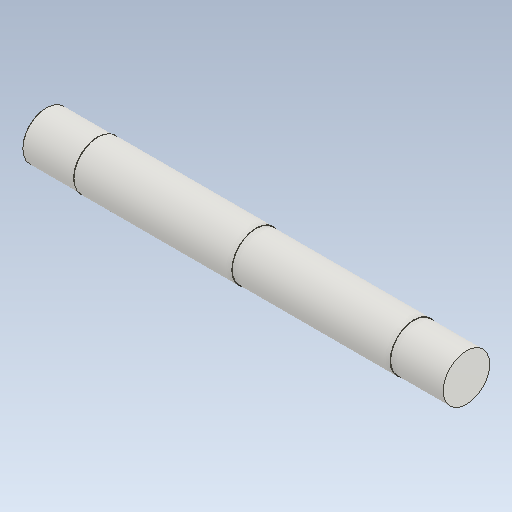
# Autodesk Inventor part: Shaft
Saved by Autodesk Inventor 2020 (Build 240168000, 168)
## iProperties
Created: 2020-11-30
Part Number: Shaft
Material: Steel
Document SubType Name: Modeling
Designer: Daniel
Density: 1 g/cm^3
Appearance: Steel
CustomPartVersion: 1
Author: Daniel
Length: 40.000 in
Autodesk Inventor part; units mm, degrees
ref_plane "Start Plane" through (0, 0, 0) normal (1, 0, 0) x (0, 1, 0)
ref_plane "XZ Plane" through (0, 0, 0) normal (0, 1, 0) x (-1, 0, 0)
ref_plane "XY Plane" through (0, 0, 0) normal (0, 0, 1) x (1, 0, 0)
sketch "Main Sketch" plane through (0, 0, 0) normal (0, 0, 1) x (1, 0, 0)
  line L0 (0, 0) -> (1016, 0)
  line L1 (0, 0) -> (0, 57.277)
  line L2 (0, 57.277) -> (127, 57.277)
  line L3 (127, 57.277) -> (127, 58.42)
  line L4 (508, 58.42) -> (508, 57.277)
  line L5 (127, 58.42) -> (508, 58.42)
  line L6 (889, 57.277) -> (889, 56.134)
  line L7 (508, 57.277) -> (889, 57.277)
  line L8 (1016, 56.134) -> (1016, 0)
  line L9 (889, 56.134) -> (1016, 56.134)
  dimension "d3" = 114.554
  dimension "d4" = 116.84
  dimension "d5" = 114.554
  dimension "d6" = 112.268
  constraints: 20 end point, 6 horizontal, 5 vertical
  measures "d3" diameter of L2 L0
  measures "d4" diameter of L5 L0
  measures "d5" diameter of L7 L0
  measures "d6" diameter of L9 L0
revolve "Revolution1" add sketch "Main Sketch" angle 360 about axis through (0, 0, 0) along (1, 0, 0)
chamfer "Chamfer1" distance 2.54 angle 45 1 edges at (0, -57.277, 0) measured on face at (0.5, -57.277, 0)
fillet "Fillet1" radius 2.54 1 edges at (127, -57.277, 0)
equation "\"Length\" = 1016"
body "Solid1"
